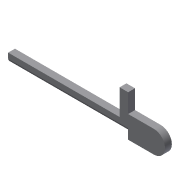
# Autodesk Inventor part: Arms
Saved by Autodesk Inventor 2018 (Build 220112000, 112)
## iProperties
Created: 2018-09-24
Part Number: Arms
Material: Generic
Document SubType Name: Modeling
Designer: DCCUMD
Density: 1 g/cm^3
Appearance: Default
Author: DCCUMD
Autodesk Inventor part; units mm, degrees
ref_plane "YZ Plane" through (0, 0, 0) normal (1, 0, 0) x (0, 1, 0)
ref_plane "XZ Plane" through (0, 0, 0) normal (0, 1, 0) x (-1, 0, 0)
ref_plane "XY Plane" through (0, 0, 0) normal (0, 0, 1) x (1, 0, 0)
sketch "Sketch1" plane through (0, 0, 0) normal (0, 1, 0) x (-1, 0, 0)
  circle A0 centre (0, 0) radius 6.5
  line L0 (0, 6.5) -> (15, 6.5)
  line L1 (15, 6.5) -> (15, -6.5)
  line L2 (15, -6.5) -> (0, -6.5)
  line L3 (0, -6.5) -> (0, 6.5)
  line L4 (15, 2.5) -> (85, 2.5)
  line L5 (85, 2.5) -> (85, -2.5)
  line L6 (85, -2.5) -> (15, -2.5)
  line L7 (15, -2.5) -> (15, 2.5)
  dimension "d0" = 13
  dimension "d1" = 6.5
  dimension "d2" = 15
  dimension "d3" = 6.5
  dimension "d4" = 70
  dimension "d5" = 4
  dimension "d6" = 4
  constraints: 16 end point, 4 parallel, 2 horizontal, 2 perpendicular, 1 coincident, 1 point on line, 1 vertical alignment, 2 other
  measures "d1" distance from line of point (0, 0) L0
  measures "d2" distance between parallel lines of L3 L1
  measures "d3" distance from line of point (0, 0) L2
  measures "d4" distance between parallel lines of L1 L5
  measures "d5" distance between parallel lines of L2 L6
  measures "d6" distance between parallel lines of L4 L0
extrude "Extrusion1" add sketch "Sketch1" along normal blind 4
fillet "Fillet1" radius 2 2 edges at (-50, 4, -2.5) (-50, 0, -2.5)
sketch "Sketch2" plane through (-85, 0, 2.5) normal (0, 0, 1) x (1, 0, 0)
  line L0 (70, 0) -> (70, 4) projected
  line L1 (0, 4) -> (70, 4) projected
  line L2 (70, 0) -> (65, 0)
  line L3 (65, 0) -> (65, 4)
  line L4 (65, 4) -> (70, 4)
  line L5 (70, 4) -> (70, 0)
  point P0 (85, 0)
  dimension "d10" = 5
  constraints: 8 end point, 2 parallel, 1 horizontal, 1 perpendicular, 1 point on line
  measures "d10" distance of L0.end L3.end
extrude "Extrusion2" add sketch "Sketch2" along normal blind 15
body "Solid1"
